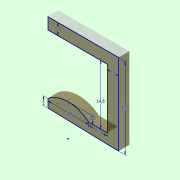
# Autodesk Inventor part: Cuvette_retainer
Saved by Autodesk Inventor 2015 (Build 190159000, 159)
## iProperties
Created: 2015-05-25
Part Number: Cuvette_retainer
Material: Generic
Document SubType Name: Modeling
Designer: Openlab
Density: 1 g/cm^3
Appearance: Polycarbonate - Smoked
Author: Openlab
Autodesk Inventor part; units mm, degrees
ref_plane "YZ Plane" through (0, 0, 0) normal (1, 0, 0) x (0, 1, 0)
ref_plane "XZ Plane" through (0, 0, 0) normal (0, 1, 0) x (-1, 0, 0)
ref_plane "XY Plane" through (0, 0, 0) normal (0, 0, 1) x (1, 0, 0)
sketch "Sketch1" plane through (0, 0, 0) normal (0, 1, 0) x (-1, 0, 0)
  line L0 (0, 0) -> (17.3, 0)
  line L1 (17.3, 0) -> (17.3, -2.8)
  line L2 (0, 0) -> (0, -19.8)
  line L3 (7.3, -17.3) -> (2.8, -17.3)
  line L4 (2.8, -17.3) -> (2.8, -2.8)
  line L5 (2.8, -2.8) -> (17.3, -2.8)
  arc A0 (17.3, -17.3) -> (7.3, -17.3) centre (12.3, -23.3444) ccw
  line L6 (7.3, -17.3) -> (18.5004, -17.3) construction
  line L7 (17.3, -17.3) -> (17.3, -19.3)
  line L8 (17.3, -19.3) -> (0, -19.8)
  point P0 (12.3, -15.5)
  dimension "d1" = 2.8
  dimension "d3" = 2.8
  dimension "d11" = 10
  dimension "d12" = 4.5
  dimension "d13" = 14.5
  dimension "d19" = 2
  dimension "d20" = 19.8
  dimension "d22" = 1.8
  constraints: 18 end point, 3 point on circle, 2 collinear, 2 perpendicular, 2 vertical, 1 centre point, 1 horizontal, 1 parallel, 1 point on line
  measures "d1" distance of L0.end L1.end
  measures "d3" distance between parallel lines of L2 L4
  measures "d11" distance of L3.start L7.start
  measures "d12" distance of L3.start L3.end
  measures "d13" distance of L3.end L4.end
  measures "d19" distance of L7.start L7.end
  measures "d20" distance of L0.start L2.end
  measures "d22" distance from line of L6 point (12.3, -15.5)
extrude "Extrusion1" add sketch "Sketch1" along normal blind 2.6
body "Solid1"
